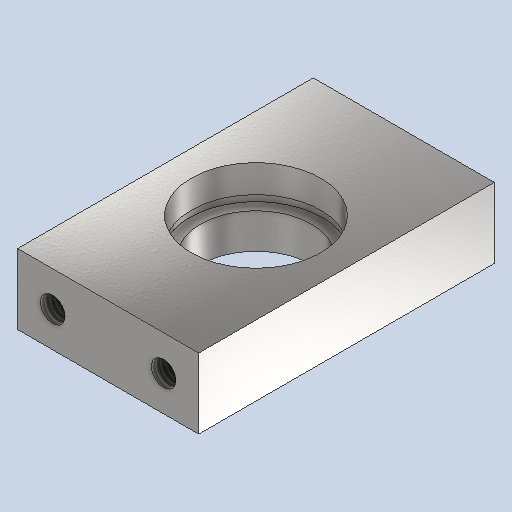
# Autodesk Inventor part: Lagerbock
Saved by Autodesk Inventor 2024 (Build 280153000, 153)
## iProperties
Created: 2024-02-29
Part Number: Lagerbock
Material: Stahl, galvanisiert
Document SubType Name: Modeling
Designer: ffogue
Density: 7.85 g/cm^3
Appearance: Galvanisiert
Author: ffogue
Autodesk Inventor part; units mm, degrees
ref_plane "YZ Plane" through (0, 0, 0) normal (1, 0, 0) x (0, 1, 0)
ref_plane "XZ Plane" through (0, 0, 0) normal (0, 1, 0) x (-1, 0, 0)
sketch "Skizze1" plane through (0, 0, 0) normal (0, 0, 1) x (1, 0, 0)
  line L0 (0, 0) -> (49, 0)
  line L1 (49, 0) -> (49, 80)
  line L2 (49, 80) -> (0, 80)
  line L3 (0, 80) -> (0, 0)
  dimension "d0" = 49
  dimension "d1" = 80
  constraints: 8 end point, 2 parallel, 1 horizontal, 1 perpendicular
  measures "d0" distance between parallel lines of L1 L3
  measures "d1" distance between parallel lines of L0 L2
extrude "Extrusion1" add sketch "Skizze1" along normal blind 19
sketch "Skizze2" plane through (0, 80, 0) normal (0, 1, 0) x (1, 0, 0)
  line L0 (0, 0) -> (0, -19) projected
  point P0 (7, -9.5)
  point P1 (0, -9.5)
  point P2 (42, -9.5)
  dimension "d11" = 7
  dimension "d12" = 35
  constraints: 1 horizontal alignment, 1 midpoint
  measures "d11" distance from line of point (7, -9.5) L0
  measures "d12" distance of point (42, -9.5) point (7, -9.5)
hole "Bohrung1" at (7, 80, 9.5) at (42, 80, 9.5) direction (0, -1, 0) diameter 4.917 depth 17.1 tip angle 118 thread size "M6x1" class "6H" standard "ISO Metric profile"
sketch "Skizze3" plane through (0, 0, 0) normal (0, -1, 0) x (1, 0, 0)
  line L0 (0, 0) -> (0, 19) projected
  point P0 (9.5, 9.5)
  point P1 (0, 9.5)
  point P2 (0, 9.5)
  point P3 (0, 9.5)
  point P4 (39.5, 9.5)
  dimension "d20" = 9.5
  dimension "d21" = 30
  constraints: 3 midpoint, 2 horizontal alignment
  measures "d20" distance of point (0, 9.5) point (9.5, 9.5)
  measures "d21" distance of point (39.5, 9.5) point (9.5, 9.5)
hole "Bohrung2" at (9.5, 0, 9.5) at (39.5, 0, 9.5) direction (0, 1, 0) diameter 6.647 depth 22.2 tip angle 118 thread size "M8x1.25" class "6H" standard "ISO Metric profile"
ref_plane "Arbeitsebene1" through (0, 0, 9.5) normal (0, 0, 1) x (1, 0, 0)
sketch "Skizze6" plane through (0, 0, 9.5) normal (0, 0, 1) x (1, 0, 0)
  line L0 (49, 0) -> (49, 80) projected
  line L1 (49, 80) -> (0, 80) projected
  point P0 (0, 0)
  point P1 (24.5, 40)
  point P2 (49, 40)
  point P3 (24.5, 80)
  constraints: 2 midpoint, 1 horizontal alignment, 1 vertical alignment
hole "Bohrung4" at (24.5, 40, 9.5) direction (0, 0, 1) diameter 35 end through all counterbore diameter 36 counterbore depth 2
hole "Bohrung5" at (24.5, 40, 9.5) direction (0, 0, -1) diameter 30 end through all
